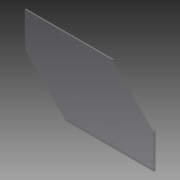
# Autodesk Inventor part: Hopper Left Side
Saved by Autodesk Inventor 2014 SP1 (Build 180222100, 222)
## iProperties
Created: 2013-12-16
Part Number: Hopper Left Side
Material: Polycarbonate, Clear
Document SubType Name: Modeling
Designer: Moses
Mass: 243.173 g
Surface Area: 1314.83 cm^2
Volume: 202.644 cm^3
Density: 1.2 g/cm^3
Appearance: Polycarbonate - Clear
Author: Moses
Autodesk Inventor part; units mm, degrees
ref_plane "YZ Plane" through (0, 0, 0) normal (1, 0, 0) x (0, 1, 0)
ref_plane "XZ Plane" through (0, 0, 0) normal (0, 1, 0) x (-1, 0, 0)
ref_plane "XY Plane" through (0, 0, 0) normal (0, 0, 1) x (1, 0, 0)
sketch "Sketch1" plane through (0, 0, 0) normal (0, 0, 1) x (1, 0, 0)
  line L0 (0, 0) -> (330.2, 0)
  line L1 (330.2, 0) -> (330.2, 193.675)
  line L2 (330.2, 193.675) -> (0, 193.675)
  line L3 (0, 193.675) -> (0, 0)
  circle A0 centre (234.95, 186.1344) radius 1.5875 projected
  circle A1 centre (95.25, 186.1344) radius 1.5875 projected
  circle A2 centre (25.4, 186.1344) radius 1.5875 projected
  circle A3 centre (165.1, 186.1344) radius 1.5875 projected
  circle A4 centre (304.8, 186.1344) radius 1.5875 projected
  line L4 (19.05, 178.5937) -> (19.05, 194.4687) construction
  line L5 (19.05, 178.5937) -> (311.15, 178.5937) construction
  line L6 (311.15, 194.4687) -> (311.15, 178.5937) construction
  line L7 (19.05, 194.4687) -> (311.15, 194.4687) construction
  circle A5 centre (115.0937, -106.3625) radius 2.54 construction
  circle A6 centre (26.1937, -106.3625) radius 2.54 construction
  circle A7 centre (219.8687, 6.35) radius 1.5875 projected
  circle A8 centre (124.6187, 6.35) radius 1.5875 projected
  circle A9 centre (29.3687, 6.35) radius 1.5875 projected
  circle A10 centre (219.8687, 44.45) radius 1.5875 projected
  circle A11 centre (124.6187, 44.45) radius 1.5875 projected
  circle A12 centre (29.3687, 44.45) radius 1.5875 projected
  line L8 (127.7937, -114.3) -> (127.7937, -88.9) construction
  line L9 (127.7937, -88.9) -> (146.8437, -88.9) construction
  line L10 (146.8437, -88.9) -> (146.8437, -114.3) construction
  line L11 (146.8437, -114.3) -> (296.0687, -114.3) construction
  line L12 (296.0687, -114.3) -> (226.2187, 0) construction
  line L13 (226.2187, 0) -> (226.2187, 50.8) construction
  line L14 (226.2187, 50.8) -> (16.6687, 50.8) construction
  line L15 (16.6687, 50.8) -> (16.6687, -114.3) construction
  line L16 (16.6687, -114.3) -> (127.7937, -114.3) construction
  circle A13 centre (7.5406, 98.425) radius 1.5875 projected
  circle A14 centre (7.5406, 15.875) radius 1.5875 projected
  circle A15 centre (7.5406, 180.975) radius 1.5875 projected
  line L17 (15.0812, 3.175) -> (-0.7937, 3.175) construction
  line L18 (15.0812, 3.175) -> (15.0812, 193.675) construction
  line L19 (-0.7937, 193.675) -> (15.0812, 193.675) construction
  line L20 (-0.7937, 3.175) -> (-0.7937, 193.675) construction
  circle A16 centre (322.6594, 15.875) radius 1.5875 projected
  circle A17 centre (322.6594, 79.375) radius 1.5875 projected
  line L21 (330.9938, 6.35) -> (315.1188, 6.35) construction
  line L22 (330.9938, 6.35) -> (330.9938, 88.9) construction
  line L23 (315.1188, 88.9) -> (330.9938, 88.9) construction
  line L24 (315.1188, 6.35) -> (315.1188, 88.9) construction
  dimension "d0" = 330.2
  dimension "d1" = 193.675
  constraints: 8 end point, 2 parallel, 1 horizontal, 1 perpendicular
  measures "d0" distance of L2.end L1.end
  measures "d1" distance of L1.end L0.end
extrude "Extrusion1" add sketch "Sketch1" along normal blind 3.175
body "Solid1"
